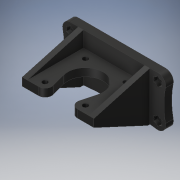
# Autodesk Inventor part: Y Motor Mount
Saved by Autodesk Inventor 2020.2 (Build 242310000, 310)
## iProperties
Created: 2018-06-16
Part Number: Y Motor Mount
Material: ABS Plastic
Document SubType Name: Modeling
Designer: Richard
Density: 1.06 g/cm^3
Appearance: Satin - Black
Author: Richard
Autodesk Inventor part; units mm, degrees
ref_plane "YZ Plane" through (0, 0, 0) normal (1, 0, 0) x (0, 1, 0)
ref_plane "XZ Plane" through (0, 0, 0) normal (0, 1, 0) x (-1, 0, 0)
ref_plane "XY Plane" through (0, 0, 0) normal (0, 0, 1) x (1, 0, 0)
sketch "Sketch1" plane through (0, 0, 0) normal (0, 0, 1) x (1, 0, 0)
  line L0 (-33.5, -13) -> (33.5, -13) construction
  line L1 (33.5, -13) -> (33.5, 13) construction
  line L2 (33.5, 13) -> (-33.5, 13) construction
  line L3 (-33.5, 13) -> (-33.5, -13) construction
  line L4 (-33.5, -13) -> (33.5, 13) construction
  line L5 (33.5, -13) -> (-33.5, 13) construction
  arc A0 (-33.5, 19) -> (-39.3825, 11.8182) centre (-33.5, 13) ccw
  arc A1 (-39.3825, -11.8182) -> (-33.5, -19) centre (-33.5, -13) ccw
  arc A2 (33.5, -19) -> (39.3825, -11.8182) centre (33.5, -13) ccw
  arc A3 (39.3825, 11.8182) -> (33.5, 19) centre (33.5, 13) ccw
  arc A4 (-39.3825, -11.8182) -> (-39.3825, 11.8182) centre (-98.207, 0) ccw
  arc A5 (39.3825, 11.8182) -> (39.3825, -11.8182) centre (98.207, 0) ccw
  line L6 (-33.5, 19) -> (33.5, 19)
  line L7 (-33.5, -19) -> (33.5, -19)
  point P0 (0, 0)
  dimension "d0" = 67
  dimension "d1" = 26
  dimension "d2" = 6
  dimension "d3" = 60
  constraints: 16 end point, 12 point on circle, 7 tangent, 6 centre point, 4 coincident, 4 equal radius, 2 horizontal, 2 midpoint, 2 parallel, 1 perpendicular
  measures "d0" distance of L1.end L2.end
  measures "d1" distance of L2.end L0.start
  measures "d2" radius of A0
  measures "d3" radius of A4
extrude "Extrusion1" add sketch "Sketch1" along normal blind 6
sketch "Sketch2" plane through (0, 0, 0) normal (1, 0, 0) x (0, 1, 0)
  line L0 (19, 6) -> (11.8182, 6) construction
  line L1 (19, 6) -> (7, 49)
  line L2 (7, 49) -> (1, 49)
  line L3 (1, 49) -> (-19, 6)
  line L4 (19, 6) -> (11.8182, 6) construction
  line L5 (11.8182, 6) -> (-11.8182, 6) construction
  line L6 (-11.8182, 6) -> (-19, 6) construction
  line L7 (-19, 6) -> (-11.8182, 6) construction
  line L8 (-11.8182, 6) -> (11.8182, 6) construction
  line L9 (11.8182, 6) -> (19, 6) construction
  line L10 (19, 6) -> (-19, 6)
  point P0 (0, 0)
  dimension "d7" = 12
  dimension "d8" = 43
  dimension "d9" = 6
  constraints: 8 end point, 1 coincident, 1 horizontal
  measures "d7" horizontal distance of L0.start L1.end
  measures "d8" distance from line of L0 L1.end
  measures "d9" distance of L1.end L2.end
extrude "Extrusion2" add sketch "Sketch2" along normal mid plane 55
sketch "Sketch3" plane through (-27.5, 1, 49) normal (0, 0, 1) x (1, 0, 0)
  line L0 (0, 0) -> (55, 0) projected
  line L1 (55, 6) -> (55, 0) projected
  line L2 (0, 6) -> (55, 6) projected
  line L3 (0, 0) -> (0, 6) projected
  line L4 (0, 6) -> (55, 6) projected
  line L5 (61, 18) -> (-6, 18) projected
  line L6 (4, 6) -> (51, 6)
  line L7 (51, 6) -> (51, 18)
  line L8 (51, 18) -> (4, 18)
  line L9 (4, 18) -> (4, 6)
  line L10 (0, 0) -> (55, 0) projected
  line L11 (-6, -20) -> (61, -20) projected
  line L12 (4, 0) -> (51, 0)
  line L13 (51, 0) -> (51, -20)
  line L14 (51, -20) -> (4, -20)
  line L15 (4, -20) -> (4, 0)
  point P0 (27.5, -1)
  dimension "d12" = 4
  dimension "d13" = 4
  constraints: 16 end point, 6 point on line, 4 parallel, 2 horizontal, 2 perpendicular
  measures "d12" distance between parallel lines of L1 L7
  measures "d13" distance between parallel lines of L3 L9
extrude "Extrusion3" cut sketch "Sketch3" against normal up to surface (43 mm away) contours L0 L13 L11 L15 | L9 L5 L7 L2
sketch "Sketch4" plane through (-23.5, 7, 49) normal (0, 1, 0) x (1, 0, 0)
  arc A0 (36.54, 17.5059) -> (10.46, 17.5059) centre (23.5, 21) ccw
  line L0 (47, 43) -> (0, 43) projected
  line L1 (57, 49) -> (-10, 49) projected
  line L2 (36.54, 17.5059) -> (31.8493, 0)
  line L3 (31.8493, 0) -> (15.1507, 0)
  line L4 (15.1507, 0) -> (10.46, 17.5059)
  line L5 (0, 0) -> (47, 0) projected
  arc A1 (10.46, 17.5059) -> (36.54, 17.5059) centre (23.5, 21) ccw construction
  point P0 (23.5, 49)
  point P1 (23.5, 49)
  point P2 (23.5, 0)
  point P3 (23.5, 49)
  dimension "d16" = 27
  dimension "d17" = 22
  dimension "d18" = 30
  constraints: 6 end point, 4 point on circle, 3 midpoint, 2 centre point, 2 vertical alignment, 1 collinear, 1 equal length, 1 horizontal, 1 tangent
  measures "d16" diameter of A0
  measures "d17" distance from line of L0 A0.centre
  measures "d18" angle of L4 L2
extrude "Extrusion4" cut sketch "Sketch4" against normal blind 55
fillet "Fillet1" radius 5 2 edges at (8.3493, 4, 49) (-8.3493, 4, 49)
sketch "Sketch5" plane through (-23.5, 7, 6) normal (0, 1, 0) x (1, 0, 0)
  arc A0 (36.54, -25.4941) -> (10.46, -25.4941) centre (23.5, -22) ccw projected
  line L0 (8, -6.5) -> (39, -6.5)
  line L1 (39, -6.5) -> (39, -37.5)
  line L2 (39, -37.5) -> (8, -37.5)
  line L3 (8, -37.5) -> (8, -6.5)
  line L4 (8, -6.5) -> (39, -37.5) construction
  line L5 (39, -6.5) -> (8, -37.5) construction
  point P0 (23.5, 6)
  dimension "d22" = 31
  dimension "d23" = 31
  constraints: 12 end point, 2 midpoint, 2 parallel, 1 horizontal, 1 perpendicular
  measures "d22" distance of L1.end L2.end
  measures "d23" distance of L0.end L1.end
hole "Hole1" at (-15.5, 7, 12.5) at (15.5, 7, 12.5) at (15.5, 7, 43.5) at (-15.5, 7, 43.5) direction (0, -1, 0) diameter 4 end through all
sketch "Sketch6" plane through (0, 0, 0) normal (0, 0, -1) x (-1, 0, 0)
  arc A0 (-33.5, -19) -> (-32.6299, -18.9366) centre (-33.5, -13) ccw
  arc A1 (32.6299, -18.9366) -> (-32.6299, -18.9366) centre (0, -241.558) ccw
  arc A2 (32.6299, -18.9366) -> (33.5, -19) centre (33.5, -13) ccw
  line L0 (-33.5, -19) -> (33.5, -19)
  arc A3 (33.5, -19) -> (39.3825, -11.8182) centre (33.5, -13) ccw projected
  arc A4 (-39.3825, -11.8182) -> (-33.5, -19) centre (-33.5, -13) ccw projected
  point P0 (0, 0)
  dimension "d31" = 225
  constraints: 6 point on circle, 4 tangent, 3 centre point, 2 concentric, 2 end point
  measures "d31" radius of A1
extrude "Extrusion5" cut sketch "Sketch6" against normal blind 55
sketch "Sketch7" plane through (0, 0, 0) normal (0, 0, -1) x (-1, 0, 0)
  line L0 (-33.5, -13) -> (33.5, -13) construction
  line L1 (33.5, -13) -> (33.5, 13) construction
  line L2 (33.5, 13) -> (-33.5, 13) construction
  line L3 (-33.5, 13) -> (-33.5, -13) construction
  line L4 (-33.5, -13) -> (33.5, 13) construction
  line L5 (33.5, -13) -> (-33.5, 13) construction
  arc A0 (-39.3825, -11.8182) -> (-32.6299, -18.9366) centre (-33.5, -13) ccw construction
  arc A1 (32.6299, -18.9366) -> (-32.6299, -18.9366) centre (0, -241.558) ccw construction
  arc A2 (32.6299, -18.9366) -> (39.3825, -11.8182) centre (33.5, -13) ccw construction
  arc A3 (39.3825, 11.8182) -> (39.3825, -11.8182) centre (98.207, 0) ccw construction
  arc A4 (39.3825, 11.8182) -> (33.5, 19) centre (33.5, 13) ccw construction
  line L6 (-33.5, 19) -> (33.5, 19) construction
  arc A5 (-33.5, 19) -> (-39.3825, 11.8182) centre (-33.5, 13) ccw construction
  arc A6 (-39.3825, -11.8182) -> (-39.3825, 11.8182) centre (-98.207, 0) ccw construction
  point P0 (0, 0)
  point P1 (0, 0)
  dimension "d34" = 67
  dimension "d35" = 26
  constraints: 12 end point, 5 coincident, 2 midpoint, 2 parallel, 1 horizontal, 1 perpendicular
  measures "d34" distance of L2.end L1.end
  measures "d35" distance of L1.end L0.end
hole "Hole2" at (33.5, 13, 0) at (33.5, -13, 0) at (-33.5, -13, 0) at (-33.5, 13, 0) direction (0, 0, 1) diameter 4 depth 14.2 tip angle 118
sketch "Sketch8" plane through (0, 0, 6) normal (0, 0, 1) x (1, 0, 0)
  circle A0 centre (-33.5, -13) radius 2 projected
  circle A1 centre (-33.5, 13) radius 2 projected
  arc A2 (-39.3825, -11.8182) -> (-32.6299, -18.9366) centre (-33.5, -13) ccw projected
  arc A3 (-27.5, -18.2449) -> (-32.6299, -18.9366) centre (0, -241.558) ccw projected
  line L0 (-27.5, -18.2449) -> (-27.5, 19) projected
  line L1 (-27.5, 19) -> (-33.5, 19) projected
  arc A4 (-33.5, 19) -> (-39.3825, 11.8182) centre (-33.5, 13) ccw projected
  arc A5 (-39.3825, -11.8182) -> (-39.3825, 11.8182) centre (-98.207, 0) ccw projected
  circle A6 centre (33.5, 13) radius 2 projected
  circle A7 centre (33.5, -13) radius 2 projected
  arc A8 (32.6299, -18.9366) -> (39.3825, -11.8182) centre (33.5, -13) ccw projected
  arc A9 (39.3825, 11.8182) -> (39.3825, -11.8182) centre (98.207, 0) ccw projected
  arc A10 (39.3825, 11.8182) -> (33.5, 19) centre (33.5, 13) ccw projected
  line L2 (33.5, 19) -> (27.5, 19) projected
  line L3 (27.5, 19) -> (27.5, -18.2449) projected
  arc A11 (32.6299, -18.9366) -> (27.5, -18.2449) centre (0, -241.558) ccw projected
  line L4 (-30.1519, 11.067) -> (-33.5, 9.134)
  line L5 (-33.5, 9.134) -> (-36.8481, 11.067)
  line L6 (-36.8481, 11.067) -> (-36.8481, 14.933)
  line L7 (-36.8481, 14.933) -> (-33.5, 16.866)
  line L8 (-33.5, 16.866) -> (-30.1519, 14.933)
  line L9 (-30.1519, 14.933) -> (-30.1519, 11.067)
  line L10 (-30.1519, -14.933) -> (-33.5, -16.866)
  line L11 (-33.5, -16.866) -> (-36.8481, -14.933)
  line L12 (-36.8481, -14.933) -> (-36.8481, -11.067)
  line L13 (-36.8481, -11.067) -> (-33.5, -9.134)
  line L14 (-33.5, -9.134) -> (-30.1519, -11.067)
  line L15 (-30.1519, -11.067) -> (-30.1519, -14.933)
  line L16 (36.8481, -14.933) -> (33.5, -16.866)
  line L17 (33.5, -16.866) -> (30.1519, -14.933)
  line L18 (30.1519, -14.933) -> (30.1519, -11.067)
  line L19 (30.1519, -11.067) -> (33.5, -9.134)
  line L20 (33.5, -9.134) -> (36.8481, -11.067)
  line L21 (36.8481, -11.067) -> (36.8481, -14.933)
  line L22 (36.8481, 11.067) -> (33.5, 9.134) construction
  line L23 (33.5, 9.134) -> (30.1519, 11.067) construction
  line L24 (30.1519, 11.067) -> (30.1519, 14.933) construction
  line L25 (30.1519, 14.933) -> (33.5, 16.866) construction
  line L26 (33.5, 16.866) -> (36.8481, 14.933) construction
  line L27 (36.8481, 14.933) -> (36.8481, 11.067) construction
  arc A12 (30.1519, 14.933) -> (33.5, 16.866) centre (30.075, 18.9323) ccw
  arc A13 (33.5, 16.866) -> (36.8481, 14.933) centre (36.925, 18.9323) ccw
  arc A14 (36.8481, 11.067) -> (33.5, 9.134) centre (36.925, 7.0677) ccw
  arc A15 (33.5, 9.134) -> (30.1519, 11.067) centre (30.075, 7.0677) ccw
  arc A16 (30.1519, 11.067) -> (30.1519, 14.933) centre (26.65, 13) ccw
  arc A17 (36.8481, 14.933) -> (36.8481, 11.067) centre (40.35, 13) ccw
  point P0 (0, 0)
  dimension "d44" = 6.6962
  dimension "d47" = 4
  dimension "d48" = 4
  dimension "d49" = 4
  dimension "d50" = 4
  dimension "d51" = 4
  dimension "d52" = 4
  dimension "d53" = 5.7
  constraints: 48 end point, 12 point on circle, 6 centre point, 4 coincident, 3 equal length, 2 point on line, 2 vertical, 52 other
  measures "d44" distance between parallel lines of L24 L27
  measures "d47" radius of A12
  measures "d48" radius of A13
  measures "d49" radius of A14
  measures "d50" radius of A15
  measures "d51" radius of A16
  measures "d52" radius of A17
extrude "Extrusion6" cut sketch "Sketch8" against normal blind 3 contours A12 A13 A17 A14 A15 A16
pattern_linear "Rectangular Pattern1" count 2 spacing 67 along (-1, 0, 0) count 2 spacing 26 along (0, -1, 0) of "Extrusion6"
equation "\"d13\" = d12"
body "Solid1"
